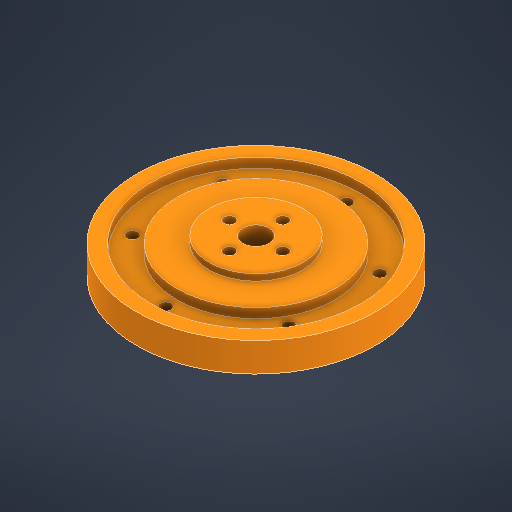
# Autodesk Inventor part: Joint - Primer segmento
Saved by Autodesk Inventor 2026 (Build 300175050, 175E)
## iProperties
Created: 2025-07-31
Part Number: Joint - Primer segmento
Material: Plastico PETG
Document SubType Name: Modeling
Designer: bello
Density: 1.27 g/cm^3
Appearance: Naranja
Author: bello
Autodesk Inventor part; units mm, degrees
ref_plane "YZ Plane" through (0, 0, 0) normal (1, 0, 0) x (0, 1, 0)
ref_plane "XZ Plane" through (0, 0, 0) normal (0, 1, 0) x (-1, 0, 0)
ref_plane "XY Plane" through (0, 0, 0) normal (0, 0, 1) x (1, 0, 0)
sketch "Boceto1" plane through (0, 0, 0) normal (0, 1, 0) x (-1, 0, 0)
  circle A0 centre (0, 0) radius 37
  dimension "d0" = 74
  constraints: 1 centre point, 1 coincident
  measures "d0" diameter of A0
extrude "Extrusión1" add sketch "Boceto1" along normal blind 11
sketch "Boceto3" plane through (0, 0, 0) normal (0, -1, 0) x (1, 0, 0)
  circle A0 centre (0, 0) radius 8.25
  circle A1 centre (0, 8.25) radius 1.7
  circle A2 centre (8.25, 0) radius 1.7
  circle A3 centre (-8.25, 0) radius 1.7
  circle A4 centre (0, -8.25) radius 1.7
  dimension "d7" = 3.4
  dimension "d8" = 16.5
  constraints: 5 centre point, 4 point on circle, 3 equal radius, 1 coincident
  measures "d7" diameter of A1
  measures "d8" diameter of A0
extrude "Extrusión3" cut sketch "Boceto3" against normal through all contours A0 A2 | A0 A2 | A1 A0 | A0 A1 | A4 A0 | A0 A4 | A3 A0 | A0 A3
sketch "Boceto5" plane through (0, 0, 0) normal (0, -1, 0) x (1, 0, 0)
  circle A0 centre (0, 0) radius 4.05
  dimension "d13" = 8.1
  constraints: 1 centre point, 1 coincident
  measures "d13" diameter of A0
extrude "Extrusión5" cut sketch "Boceto5" against normal through all
sketch "Boceto8" plane through (0, 11, 0) normal (0, 1, 0) x (1, 0, 0)
  circle A0 centre (0, 0) radius 24.5
  circle A1 centre (0, 0) radius 37
  dimension "d25" = 49
  dimension "d26" = 74
  constraints: 2 centre point, 2 coincident
  measures "d25" diameter of A0
  measures "d26" diameter of A1
extrude "Extrusión8" cut sketch "Boceto8" against normal blind 2
sketch "Boceto14" plane through (0, 9, 0) normal (0, 1, 0) x (1, 0, 0)
  circle A0 centre (0, 0) radius 28
  circle A1 centre (0, 28) radius 1.7
  circle A2 centre (-24.2487, 14) radius 1.7
  circle A3 centre (-24.2487, -14) radius 1.7
  circle A4 centre (0, -28) radius 1.7
  circle A5 centre (24.2487, -14) radius 1.7
  circle A6 centre (24.2487, 14) radius 1.7
  point P0 (-1.6992, -27.9484)
  point P1 (1.6992, -27.9484)
  dimension "d50" = 56
  dimension "d51" = 3.4
  dimension "d54" = 360
  constraints: 6 centre point, 1 coincident, 16 other
  measures "d51" diameter of A1
extrude "Extrusión12" cut sketch "Boceto14" against normal through all contours A6 A0 | A0 A6 | A5 A0 | A0 A5 | A1 A0 | A0 A1 | A4 A0 | A0 A4 | A2 A0 | A0 A2 | A3 A0 | A0 A3
sketch "Boceto15" plane through (0, 9, 0) normal (0, 1, 0) x (1, 0, 0)
  circle A0 centre (24.2487, 14) radius 1.7 projected
  circle A1 centre (24.2487, 14) radius 3
  circle A2 centre (0, 28) radius 3
  circle A3 centre (-24.2487, 14) radius 3
  circle A4 centre (-24.2487, -14) radius 3
  circle A5 centre (0, -28) radius 3
  circle A6 centre (24.2487, -14) radius 3
  circle A7 centre (0, 0) radius 4.05 projected
  circle A8 centre (0, 0) radius 32.5
  circle A9 centre (0, 0) radius 24.5
  dimension "d58" = 6
  dimension "d61" = 360
  dimension "d63" = 65
  constraints: 8 centre point, 3 coincident, 13 other
  measures "d58" diameter of A1
  measures "d63" diameter of A8
extrude "Extrusión13" cut sketch "Boceto15" against normal blind 3 contours A0 | A1 | A2 | A3 | A4 | A5 | A6 | A8
sketch "Boceto16" plane through (0, 11, 0) normal (0, 1, 0) x (1, 0, 0)
  circle A0 centre (0, 0) radius 14.5
  circle A1 centre (0, 0) radius 37
  dimension "d66" = 29
  constraints: 2 centre point, 2 coincident
  measures "d66" diameter of A0
extrude "Extrusión14" cut sketch "Boceto16" against normal blind 2
equation "\"d1\" = Altura"
equation "\"Altura\" = 11"
